Autodesk Fusion 360 part; units mm, degrees
(part 3 of 3)
  arc A127 (-91.1567, -68.8169) -> (-88.1567, -65.8169) centre (-91.1567, -65.8169) ccw
  line L128 (-91.1567, -127.2613) -> (-95.1567, -127.2613)
  arc A128 (-98.1567, -124.2613) -> (-95.1567, -127.2613) centre (-95.1567, -124.2613) ccw
  line L129 (-98.1567, -124.2613) -> (-98.1567, -120.2613)
  arc A129 (-95.1567, -117.2613) -> (-98.1567, -120.2613) centre (-95.1567, -120.2613) ccw
  line L130 (-95.1567, -117.2613) -> (-91.1567, -117.2613)
  arc A130 (-88.1567, -120.2613) -> (-91.1567, -117.2613) centre (-91.1567, -120.2613) ccw
  line L131 (-88.1567, -120.2613) -> (-88.1567, -124.2613)
  arc A131 (-91.1567, -127.2613) -> (-88.1567, -124.2613) centre (-91.1567, -124.2613) ccw
  line L132 (-120.3789, -156.4835) -> (-124.3789, -156.4835)
  arc A132 (-127.3789, -153.4835) -> (-124.3789, -156.4835) centre (-124.3789, -153.4835) ccw
  line L133 (-127.3789, -153.4835) -> (-127.3789, -149.4835)
  arc A133 (-124.3789, -146.4835) -> (-127.3789, -149.4835) centre (-124.3789, -149.4835) ccw
  line L134 (-124.3789, -146.4835) -> (-120.3789, -146.4835)
  arc A134 (-117.3789, -149.4835) -> (-120.3789, -146.4835) centre (-120.3789, -149.4835) ccw
  line L135 (-117.3789, -149.4835) -> (-117.3789, -153.4835)
  arc A135 (-120.3789, -156.4835) -> (-117.3789, -153.4835) centre (-120.3789, -153.4835) ccw
  line L136 (-105.7678, -141.8724) -> (-109.7678, -141.8724)
  arc A136 (-112.7678, -138.8724) -> (-109.7678, -141.8724) centre (-109.7678, -138.8724) ccw
  line L137 (-112.7678, -138.8724) -> (-112.7678, -134.8724)
  arc A137 (-109.7678, -131.8724) -> (-112.7678, -134.8724) centre (-109.7678, -134.8724) ccw
  line L138 (-109.7678, -131.8724) -> (-105.7678, -131.8724)
  arc A138 (-102.7678, -134.8724) -> (-105.7678, -131.8724) centre (-105.7678, -134.8724) ccw
  line L139 (-102.7678, -134.8724) -> (-102.7678, -138.8724)
  arc A139 (-105.7678, -141.8724) -> (-102.7678, -138.8724) centre (-105.7678, -138.8724) ccw
  line L140 (-134.99, -156.4835) -> (-138.99, -156.4835)
  arc A140 (-141.99, -153.4835) -> (-138.99, -156.4835) centre (-138.99, -153.4835) ccw
  line L141 (-141.99, -153.4835) -> (-141.99, -149.4835)
  arc A141 (-138.99, -146.4835) -> (-141.99, -149.4835) centre (-138.99, -149.4835) ccw
  line L142 (-138.99, -146.4835) -> (-134.99, -146.4835)
  arc A142 (-131.99, -149.4835) -> (-134.99, -146.4835) centre (-134.99, -149.4835) ccw
  line L143 (-131.99, -149.4835) -> (-131.99, -153.4835)
  arc A143 (-134.99, -156.4835) -> (-131.99, -153.4835) centre (-134.99, -153.4835) ccw
  line L144 (-120.3789, -39.5946) -> (-124.3789, -39.5946)
  arc A144 (-127.3789, -36.5946) -> (-124.3789, -39.5946) centre (-124.3789, -36.5946) ccw
  line L145 (-127.3789, -36.5946) -> (-127.3789, -32.5946)
  arc A145 (-124.3789, -29.5946) -> (-127.3789, -32.5946) centre (-124.3789, -32.5946) ccw
  line L146 (-124.3789, -29.5946) -> (-120.3789, -29.5946)
  arc A146 (-117.3789, -32.5946) -> (-120.3789, -29.5946) centre (-120.3789, -32.5946) ccw
  line L147 (-117.3789, -32.5946) -> (-117.3789, -36.5946)
  arc A147 (-120.3789, -39.5946) -> (-117.3789, -36.5946) centre (-120.3789, -36.5946) ccw
  line L148 (-134.99, -98.0391) -> (-138.99, -98.0391)
  arc A148 (-141.99, -95.0391) -> (-138.99, -98.0391) centre (-138.99, -95.0391) ccw
  line L149 (-141.99, -95.0391) -> (-141.99, -91.0391)
  arc A149 (-138.99, -88.0391) -> (-141.99, -91.0391) centre (-138.99, -91.0391) ccw
  line L150 (-138.99, -88.0391) -> (-134.99, -88.0391)
  arc A150 (-131.99, -91.0391) -> (-134.99, -88.0391) centre (-134.99, -91.0391) ccw
  line L151 (-131.99, -91.0391) -> (-131.99, -95.0391)
  arc A151 (-134.99, -98.0391) -> (-131.99, -95.0391) centre (-134.99, -95.0391) ccw
  line L152 (-164.2123, -68.8169) -> (-168.2123, -68.8169)
  arc A152 (-171.2123, -65.8169) -> (-168.2123, -68.8169) centre (-168.2123, -65.8169) ccw
  line L153 (-171.2123, -65.8169) -> (-171.2123, -61.8169)
  arc A153 (-168.2123, -58.8169) -> (-171.2123, -61.8169) centre (-168.2123, -61.8169) ccw
  line L154 (-168.2123, -58.8169) -> (-164.2123, -58.8169)
  arc A154 (-161.2123, -61.8169) -> (-164.2123, -58.8169) centre (-164.2123, -61.8169) ccw
  line L155 (-161.2123, -61.8169) -> (-161.2123, -65.8169)
  arc A155 (-164.2123, -68.8169) -> (-161.2123, -65.8169) centre (-164.2123, -65.8169) ccw
  line L156 (-91.1567, -141.8724) -> (-95.1567, -141.8724)
  arc A156 (-98.1567, -138.8724) -> (-95.1567, -141.8724) centre (-95.1567, -138.8724) ccw
  line L157 (-98.1567, -138.8724) -> (-98.1567, -134.8724)
  arc A157 (-95.1567, -131.8724) -> (-98.1567, -134.8724) centre (-95.1567, -134.8724) ccw
  line L158 (-95.1567, -131.8724) -> (-91.1567, -131.8724)
  arc A158 (-88.1567, -134.8724) -> (-91.1567, -131.8724) centre (-91.1567, -134.8724) ccw
  line L159 (-88.1567, -134.8724) -> (-88.1567, -138.8724)
  arc A159 (-91.1567, -141.8724) -> (-88.1567, -138.8724) centre (-91.1567, -138.8724) ccw
  line L160 (-149.6011, -112.6502) -> (-153.6011, -112.6502)
  arc A160 (-156.6011, -109.6502) -> (-153.6011, -112.6502) centre (-153.6011, -109.6502) ccw
  line L161 (-156.6011, -109.6502) -> (-156.6011, -105.6502)
  arc A161 (-153.6011, -102.6502) -> (-156.6011, -105.6502) centre (-153.6011, -105.6502) ccw
  line L162 (-153.6011, -102.6502) -> (-149.6011, -102.6502)
  arc A162 (-146.6011, -105.6502) -> (-149.6011, -102.6502) centre (-149.6011, -105.6502) ccw
  line L163 (-146.6011, -105.6502) -> (-146.6011, -109.6502)
  arc A163 (-149.6011, -112.6502) -> (-146.6011, -109.6502) centre (-149.6011, -109.6502) ccw
  line L164 (-105.7678, -112.6502) -> (-109.7678, -112.6502)
  arc A164 (-112.7678, -109.6502) -> (-109.7678, -112.6502) centre (-109.7678, -109.6502) ccw
  line L165 (-112.7678, -109.6502) -> (-112.7678, -105.6502)
  arc A165 (-109.7678, -102.6502) -> (-112.7678, -105.6502) centre (-109.7678, -105.6502) ccw
  line L166 (-109.7678, -102.6502) -> (-105.7678, -102.6502)
  arc A166 (-102.7678, -105.6502) -> (-105.7678, -102.6502) centre (-105.7678, -105.6502) ccw
  line L167 (-102.7678, -105.6502) -> (-102.7678, -109.6502)
  arc A167 (-105.7678, -112.6502) -> (-102.7678, -109.6502) centre (-105.7678, -109.6502) ccw
  line L168 (-76.5456, -141.8724) -> (-80.5456, -141.8724)
  arc A168 (-83.5456, -138.8724) -> (-80.5456, -141.8724) centre (-80.5456, -138.8724) ccw
  line L169 (-83.5456, -138.8724) -> (-83.5456, -134.8724)
  arc A169 (-80.5456, -131.8724) -> (-83.5456, -134.8724) centre (-80.5456, -134.8724) ccw
  line L170 (-80.5456, -131.8724) -> (-76.5456, -131.8724)
  arc A170 (-73.5456, -134.8724) -> (-76.5456, -131.8724) centre (-76.5456, -134.8724) ccw
  line L171 (-73.5456, -134.8724) -> (-73.5456, -138.8724)
  arc A171 (-76.5456, -141.8724) -> (-73.5456, -138.8724) centre (-76.5456, -138.8724) ccw
  line L172 (-149.6011, -127.2613) -> (-153.6011, -127.2613)
  arc A172 (-156.6011, -124.2613) -> (-153.6011, -127.2613) centre (-153.6011, -124.2613) ccw
  line L173 (-156.6011, -124.2613) -> (-156.6011, -120.2613)
  arc A173 (-153.6011, -117.2613) -> (-156.6011, -120.2613) centre (-153.6011, -120.2613) ccw
  line L174 (-153.6011, -117.2613) -> (-149.6011, -117.2613)
  arc A174 (-146.6011, -120.2613) -> (-149.6011, -117.2613) centre (-149.6011, -120.2613) ccw
  line L175 (-146.6011, -120.2613) -> (-146.6011, -124.2613)
  arc A175 (-149.6011, -127.2613) -> (-146.6011, -124.2613) centre (-149.6011, -124.2613) ccw
  line L176 (-164.2123, -141.8724) -> (-168.2123, -141.8724)
  arc A176 (-171.2123, -138.8724) -> (-168.2123, -141.8724) centre (-168.2123, -138.8724) ccw
  line L177 (-171.2123, -138.8724) -> (-171.2123, -134.8724)
  arc A177 (-168.2123, -131.8724) -> (-171.2123, -134.8724) centre (-168.2123, -134.8724) ccw
  line L178 (-168.2123, -131.8724) -> (-164.2123, -131.8724)
  arc A178 (-161.2123, -134.8724) -> (-164.2123, -131.8724) centre (-164.2123, -134.8724) ccw
  line L179 (-161.2123, -134.8724) -> (-161.2123, -138.8724)
  arc A179 (-164.2123, -141.8724) -> (-161.2123, -138.8724) centre (-164.2123, -138.8724) ccw
  line L180 (-47.3234, -171.0946) -> (-51.3234, -171.0946)
  arc A180 (-54.3234, -168.0946) -> (-51.3234, -171.0946) centre (-51.3234, -168.0946) ccw
  line L181 (-54.3234, -168.0946) -> (-54.3234, -164.0946)
  arc A181 (-51.3234, -161.0946) -> (-54.3234, -164.0946) centre (-51.3234, -164.0946) ccw
  line L182 (-51.3234, -161.0946) -> (-47.3234, -161.0946)
  arc A182 (-44.3234, -164.0946) -> (-47.3234, -161.0946) centre (-47.3234, -164.0946) ccw
  line L183 (-44.3234, -164.0946) -> (-44.3234, -168.0946)
  arc A183 (-47.3234, -171.0946) -> (-44.3234, -168.0946) centre (-47.3234, -168.0946) ccw
  line L184 (-32.7123, -156.4835) -> (-36.7123, -156.4835)
  arc A184 (-39.7123, -153.4835) -> (-36.7123, -156.4835) centre (-36.7123, -153.4835) ccw
  line L185 (-39.7123, -153.4835) -> (-39.7123, -149.4835)
  arc A185 (-36.7123, -146.4835) -> (-39.7123, -149.4835) centre (-36.7123, -149.4835) ccw
  line L186 (-36.7123, -146.4835) -> (-32.7123, -146.4835)
  arc A186 (-29.7123, -149.4835) -> (-32.7123, -146.4835) centre (-32.7123, -149.4835) ccw
  line L187 (-29.7123, -149.4835) -> (-29.7123, -153.4835)
  arc A187 (-32.7123, -156.4835) -> (-29.7123, -153.4835) centre (-32.7123, -153.4835) ccw
  line L188 (-32.7123, -127.2613) -> (-36.7123, -127.2613)
  arc A188 (-39.7123, -124.2613) -> (-36.7123, -127.2613) centre (-36.7123, -124.2613) ccw
  line L189 (-39.7123, -124.2613) -> (-39.7123, -120.2613)
  arc A189 (-36.7123, -117.2613) -> (-39.7123, -120.2613) centre (-36.7123, -120.2613) ccw
  line L190 (-36.7123, -117.2613) -> (-32.7123, -117.2613)
  arc A190 (-29.7123, -120.2613) -> (-32.7123, -117.2613) centre (-32.7123, -120.2613) ccw
  line L191 (-29.7123, -120.2613) -> (-29.7123, -124.2613)
  arc A191 (-32.7123, -127.2613) -> (-29.7123, -124.2613) centre (-32.7123, -124.2613) ccw
  line L192 (-47.3234, -127.2613) -> (-51.3234, -127.2613)
  arc A192 (-54.3234, -124.2613) -> (-51.3234, -127.2613) centre (-51.3234, -124.2613) ccw
  line L193 (-54.3234, -124.2613) -> (-54.3234, -120.2613)
  arc A193 (-51.3234, -117.2613) -> (-54.3234, -120.2613) centre (-51.3234, -120.2613) ccw
  line L194 (-51.3234, -117.2613) -> (-47.3234, -117.2613)
  arc A194 (-44.3234, -120.2613) -> (-47.3234, -117.2613) centre (-47.3234, -120.2613) ccw
  line L195 (-44.3234, -120.2613) -> (-44.3234, -124.2613)
  arc A195 (-47.3234, -127.2613) -> (-44.3234, -124.2613) centre (-47.3234, -124.2613) ccw
  line L196 (-105.7678, -83.428) -> (-109.7678, -83.428)
  arc A196 (-112.7678, -80.428) -> (-109.7678, -83.428) centre (-109.7678, -80.428) ccw
  line L197 (-112.7678, -80.428) -> (-112.7678, -76.428)
  arc A197 (-109.7678, -73.428) -> (-112.7678, -76.428) centre (-109.7678, -76.428) ccw
  line L198 (-109.7678, -73.428) -> (-105.7678, -73.428)
  arc A198 (-102.7678, -76.428) -> (-105.7678, -73.428) centre (-105.7678, -76.428) ccw
  line L199 (-102.7678, -76.428) -> (-102.7678, -80.428)
  arc A199 (-105.7678, -83.428) -> (-102.7678, -80.428) centre (-105.7678, -80.428) ccw
  line L200 (-120.3789, -68.8169) -> (-124.3789, -68.8169)
  arc A200 (-127.3789, -65.8169) -> (-124.3789, -68.8169) centre (-124.3789, -65.8169) ccw
  line L201 (-127.3789, -65.8169) -> (-127.3789, -61.8169)
  arc A201 (-124.3789, -58.8169) -> (-127.3789, -61.8169) centre (-124.3789, -61.8169) ccw
  line L202 (-124.3789, -58.8169) -> (-120.3789, -58.8169)
  arc A202 (-117.3789, -61.8169) -> (-120.3789, -58.8169) centre (-120.3789, -61.8169) ccw
  line L203 (-117.3789, -61.8169) -> (-117.3789, -65.8169)
  arc A203 (-120.3789, -68.8169) -> (-117.3789, -65.8169) centre (-120.3789, -65.8169) ccw
  line L204 (-91.1567, -171.0946) -> (-95.1567, -171.0946)
  arc A204 (-98.1567, -168.0946) -> (-95.1567, -171.0946) centre (-95.1567, -168.0946) ccw
  line L205 (-98.1567, -168.0946) -> (-98.1567, -164.0946)
  arc A205 (-95.1567, -161.0946) -> (-98.1567, -164.0946) centre (-95.1567, -164.0946) ccw
  line L206 (-95.1567, -161.0946) -> (-91.1567, -161.0946)
  arc A206 (-88.1567, -164.0946) -> (-91.1567, -161.0946) centre (-91.1567, -164.0946) ccw
  line L207 (-88.1567, -164.0946) -> (-88.1567, -168.0946)
  arc A207 (-91.1567, -171.0946) -> (-88.1567, -168.0946) centre (-91.1567, -168.0946) ccw
  line L208 (-47.3234, -156.4835) -> (-51.3234, -156.4835)
  arc A208 (-54.3234, -153.4835) -> (-51.3234, -156.4835) centre (-51.3234, -153.4835) ccw
  line L209 (-54.3234, -153.4835) -> (-54.3234, -149.4835)
  arc A209 (-51.3234, -146.4835) -> (-54.3234, -149.4835) centre (-51.3234, -149.4835) ccw
  line L210 (-51.3234, -146.4835) -> (-47.3234, -146.4835)
  arc A210 (-44.3234, -149.4835) -> (-47.3234, -146.4835) centre (-47.3234, -149.4835) ccw
  line L211 (-44.3234, -149.4835) -> (-44.3234, -153.4835)
  arc A211 (-47.3234, -156.4835) -> (-44.3234, -153.4835) centre (-47.3234, -153.4835) ccw
  line L212 (-134.99, -39.5946) -> (-138.99, -39.5946)
  arc A212 (-141.99, -36.5946) -> (-138.99, -39.5946) centre (-138.99, -36.5946) ccw
  line L213 (-141.99, -36.5946) -> (-141.99, -32.5946)
  arc A213 (-138.99, -29.5946) -> (-141.99, -32.5946) centre (-138.99, -32.5946) ccw
  line L214 (-138.99, -29.5946) -> (-134.99, -29.5946)
  arc A214 (-131.99, -32.5946) -> (-134.99, -29.5946) centre (-134.99, -32.5946) ccw
  line L215 (-131.99, -32.5946) -> (-131.99, -36.5946)
  arc A215 (-134.99, -39.5946) -> (-131.99, -36.5946) centre (-134.99, -36.5946) ccw
  line L216 (-134.99, -141.8724) -> (-138.99, -141.8724)
  arc A216 (-141.99, -138.8724) -> (-138.99, -141.8724) centre (-138.99, -138.8724) ccw
  line L217 (-141.99, -138.8724) -> (-141.99, -134.8724)
  arc A217 (-138.99, -131.8724) -> (-141.99, -134.8724) centre (-138.99, -134.8724) ccw
  line L218 (-138.99, -131.8724) -> (-134.99, -131.8724)
  arc A218 (-131.99, -134.8724) -> (-134.99, -131.8724) centre (-134.99, -134.8724) ccw
  line L219 (-131.99, -134.8724) -> (-131.99, -138.8724)
  arc A219 (-134.99, -141.8724) -> (-131.99, -138.8724) centre (-134.99, -138.8724) ccw
  line L220 (-120.3789, -127.2613) -> (-124.3789, -127.2613)
  arc A220 (-127.3789, -124.2613) -> (-124.3789, -127.2613) centre (-124.3789, -124.2613) ccw
  line L221 (-127.3789, -124.2613) -> (-127.3789, -120.2613)
  arc A221 (-124.3789, -117.2613) -> (-127.3789, -120.2613) centre (-124.3789, -120.2613) ccw
  line L222 (-124.3789, -117.2613) -> (-120.3789, -117.2613)
  arc A222 (-117.3789, -120.2613) -> (-120.3789, -117.2613) centre (-120.3789, -120.2613) ccw
  line L223 (-117.3789, -120.2613) -> (-117.3789, -124.2613)
  arc A223 (-120.3789, -127.2613) -> (-117.3789, -124.2613) centre (-120.3789, -124.2613) ccw
  line L224 (-164.2123, -127.2613) -> (-168.2123, -127.2613)
  arc A224 (-171.2123, -124.2613) -> (-168.2123, -127.2613) centre (-168.2123, -124.2613) ccw
  line L225 (-171.2123, -124.2613) -> (-171.2123, -120.2613)
  arc A225 (-168.2123, -117.2613) -> (-171.2123, -120.2613) centre (-168.2123, -120.2613) ccw
  line L226 (-168.2123, -117.2613) -> (-164.2123, -117.2613)
  arc A226 (-161.2123, -120.2613) -> (-164.2123, -117.2613) centre (-164.2123, -120.2613) ccw
  line L227 (-161.2123, -120.2613) -> (-161.2123, -124.2613)
  arc A227 (-164.2123, -127.2613) -> (-161.2123, -124.2613) centre (-164.2123, -124.2613) ccw
  line L228 (-134.99, -68.8169) -> (-138.99, -68.8169)
  arc A228 (-141.99, -65.8169) -> (-138.99, -68.8169) centre (-138.99, -65.8169) ccw
  line L229 (-141.99, -65.8169) -> (-141.99, -61.8169)
  arc A229 (-138.99, -58.8169) -> (-141.99, -61.8169) centre (-138.99, -61.8169) ccw
  line L230 (-138.99, -58.8169) -> (-134.99, -58.8169)
  arc A230 (-131.99, -61.8169) -> (-134.99, -58.8169) centre (-134.99, -61.8169) ccw
  line L231 (-131.99, -61.8169) -> (-131.99, -65.8169)
  arc A231 (-134.99, -68.8169) -> (-131.99, -65.8169) centre (-134.99, -65.8169) ccw
  line L232 (-32.7123, -171.0946) -> (-36.7123, -171.0946)
  arc A232 (-39.7123, -168.0946) -> (-36.7123, -171.0946) centre (-36.7123, -168.0946) ccw
  line L233 (-39.7123, -168.0946) -> (-39.7123, -164.0946)
  arc A233 (-36.7123, -161.0946) -> (-39.7123, -164.0946) centre (-36.7123, -164.0946) ccw
  line L234 (-36.7123, -161.0946) -> (-32.7123, -161.0946)
  arc A234 (-29.7123, -164.0946) -> (-32.7123, -161.0946) centre (-32.7123, -164.0946) ccw
  line L235 (-29.7123, -164.0946) -> (-29.7123, -168.0946)
  arc A235 (-32.7123, -171.0946) -> (-29.7123, -168.0946) centre (-32.7123, -168.0946) ccw
  line L236 (-105.7678, -54.2058) -> (-109.7678, -54.2058)
  arc A236 (-112.7678, -51.2058) -> (-109.7678, -54.2058) centre (-109.7678, -51.2058) ccw
  line L237 (-112.7678, -51.2058) -> (-112.7678, -47.2058)
  arc A237 (-109.7678, -44.2058) -> (-112.7678, -47.2058) centre (-109.7678, -47.2058) ccw
  line L238 (-109.7678, -44.2058) -> (-105.7678, -44.2058)
  arc A238 (-102.7678, -47.2058) -> (-105.7678, -44.2058) centre (-105.7678, -47.2058) ccw
  line L239 (-102.7678, -47.2058) -> (-102.7678, -51.2058)
  arc A239 (-105.7678, -54.2058) -> (-102.7678, -51.2058) centre (-105.7678, -51.2058) ccw
  line L240 (-61.9345, -171.0946) -> (-65.9345, -171.0946)
  arc A240 (-68.9345, -168.0946) -> (-65.9345, -171.0946) centre (-65.9345, -168.0946) ccw
  line L241 (-68.9345, -168.0946) -> (-68.9345, -164.0946)
  arc A241 (-65.9345, -161.0946) -> (-68.9345, -164.0946) centre (-65.9345, -164.0946) ccw
  line L242 (-65.9345, -161.0946) -> (-61.9345, -161.0946)
  arc A242 (-58.9345, -164.0946) -> (-61.9345, -161.0946) centre (-61.9345, -164.0946) ccw
  line L243 (-58.9345, -164.0946) -> (-58.9345, -168.0946)
  arc A243 (-61.9345, -171.0946) -> (-58.9345, -168.0946) centre (-61.9345, -168.0946) ccw
  line L244 (-47.3234, -141.8724) -> (-51.3234, -141.8724)
  arc A244 (-54.3234, -138.8724) -> (-51.3234, -141.8724) centre (-51.3234, -138.8724) ccw
  line L245 (-54.3234, -138.8724) -> (-54.3234, -134.8724)
  arc A245 (-51.3234, -131.8724) -> (-54.3234, -134.8724) centre (-51.3234, -134.8724) ccw
  line L246 (-51.3234, -131.8724) -> (-47.3234, -131.8724)
  arc A246 (-44.3234, -134.8724) -> (-47.3234, -131.8724) centre (-47.3234, -134.8724) ccw
  line L247 (-44.3234, -134.8724) -> (-44.3234, -138.8724)
  arc A247 (-47.3234, -141.8724) -> (-44.3234, -138.8724) centre (-47.3234, -138.8724) ccw
  line L248 (-149.6011, -98.0391) -> (-153.6011, -98.0391)
  arc A248 (-156.6011, -95.0391) -> (-153.6011, -98.0391) centre (-153.6011, -95.0391) ccw
  line L249 (-156.6011, -95.0391) -> (-156.6011, -91.0391)
  arc A249 (-153.6011, -88.0391) -> (-156.6011, -91.0391) centre (-153.6011, -91.0391) ccw
  line L250 (-153.6011, -88.0391) -> (-149.6011, -88.0391)
  arc A250 (-146.6011, -91.0391) -> (-149.6011, -88.0391) centre (-149.6011, -91.0391) ccw
  line L251 (-146.6011, -91.0391) -> (-146.6011, -95.0391)
  arc A251 (-149.6011, -98.0391) -> (-146.6011, -95.0391) centre (-149.6011, -95.0391) ccw
  line L252 (-149.6011, -54.2058) -> (-153.6011, -54.2058)
  arc A252 (-156.6011, -51.2058) -> (-153.6011, -54.2058) centre (-153.6011, -51.2058) ccw
  line L253 (-156.6011, -51.2058) -> (-156.6011, -47.2058)
  arc A253 (-153.6011, -44.2058) -> (-156.6011, -47.2058) centre (-153.6011, -47.2058) ccw
  line L254 (-153.6011, -44.2058) -> (-149.6011, -44.2058)
  arc A254 (-146.6011, -47.2058) -> (-149.6011, -44.2058) centre (-149.6011, -47.2058) ccw
  line L255 (-146.6011, -47.2058) -> (-146.6011, -51.2058)
  arc A255 (-149.6011, -54.2058) -> (-146.6011, -51.2058) centre (-149.6011, -51.2058) ccw
  line L256 (-105.7678, -156.4835) -> (-109.7678, -156.4835)
  arc A256 (-112.7678, -153.4835) -> (-109.7678, -156.4835) centre (-109.7678, -153.4835) ccw
  line L257 (-112.7678, -153.4835) -> (-112.7678, -149.4835)
  arc A257 (-109.7678, -146.4835) -> (-112.7678, -149.4835) centre (-109.7678, -149.4835) ccw
  line L258 (-109.7678, -146.4835) -> (-105.7678, -146.4835)
  arc A258 (-102.7678, -149.4835) -> (-105.7678, -146.4835) centre (-105.7678, -149.4835) ccw
  line L259 (-102.7678, -149.4835) -> (-102.7678, -153.4835)
  arc A259 (-105.7678, -156.4835) -> (-102.7678, -153.4835) centre (-105.7678, -153.4835) ccw
  line L260 (-164.2123, -171.0946) -> (-168.2123, -171.0946)
  arc A260 (-171.2123, -168.0946) -> (-168.2123, -171.0946) centre (-168.2123, -168.0946) ccw
  line L261 (-171.2123, -168.0946) -> (-171.2123, -164.0946)
  arc A261 (-168.2123, -161.0946) -> (-171.2123, -164.0946) centre (-168.2123, -164.0946) ccw
  line L262 (-168.2123, -161.0946) -> (-164.2123, -161.0946)
  arc A262 (-161.2123, -164.0946) -> (-164.2123, -161.0946) centre (-164.2123, -164.0946) ccw
  line L263 (-161.2123, -164.0946) -> (-161.2123, -168.0946)
  arc A263 (-164.2123, -171.0946) -> (-161.2123, -168.0946) centre (-164.2123, -168.0946) ccw
  line L264 (-149.6011, -171.0946) -> (-153.6011, -171.0946)
  arc A264 (-156.6011, -168.0946) -> (-153.6011, -171.0946) centre (-153.6011, -168.0946) ccw
  line L265 (-156.6011, -168.0946) -> (-156.6011, -164.0946)
  arc A265 (-153.6011, -161.0946) -> (-156.6011, -164.0946) centre (-153.6011, -164.0946) ccw
  line L266 (-153.6011, -161.0946) -> (-149.6011, -161.0946)
  arc A266 (-146.6011, -164.0946) -> (-149.6011, -161.0946) centre (-149.6011, -164.0946) ccw
  line L267 (-146.6011, -164.0946) -> (-146.6011, -168.0946)
  arc A267 (-149.6011, -171.0946) -> (-146.6011, -168.0946) centre (-149.6011, -168.0946) ccw
  line L268 (-91.1567, -83.428) -> (-95.1567, -83.428)
  arc A268 (-98.1567, -80.428) -> (-95.1567, -83.428) centre (-95.1567, -80.428) ccw
  line L269 (-98.1567, -80.428) -> (-98.1567, -76.428)
  arc A269 (-95.1567, -73.428) -> (-98.1567, -76.428) centre (-95.1567, -76.428) ccw
  line L270 (-95.1567, -73.428) -> (-91.1567, -73.428)
  arc A270 (-88.1567, -76.428) -> (-91.1567, -73.428) centre (-91.1567, -76.428) ccw
  line L271 (-88.1567, -76.428) -> (-88.1567, -80.428)
  arc A271 (-91.1567, -83.428) -> (-88.1567, -80.428) centre (-91.1567, -80.428) ccw
  line L272 (-47.3234, -68.8169) -> (-51.3234, -68.8169)
  arc A272 (-54.3234, -65.8169) -> (-51.3234, -68.8169) centre (-51.3234, -65.8169) ccw
  line L273 (-54.3234, -65.8169) -> (-54.3234, -61.8169)
  arc A273 (-51.3234, -58.8169) -> (-54.3234, -61.8169) centre (-51.3234, -61.8169) ccw
  line L274 (-51.3234, -58.8169) -> (-47.3234, -58.8169)
  arc A274 (-44.3234, -61.8169) -> (-47.3234, -58.8169) centre (-47.3234, -61.8169) ccw
  line L275 (-44.3234, -61.8169) -> (-44.3234, -65.8169)
  arc A275 (-47.3234, -68.8169) -> (-44.3234, -65.8169) centre (-47.3234, -65.8169) ccw
  line L276 (-32.7123, -54.2058) -> (-36.7123, -54.2058)
  arc A276 (-39.7123, -51.2058) -> (-36.7123, -54.2058) centre (-36.7123, -51.2058) ccw
  line L277 (-39.7123, -51.2058) -> (-39.7123, -47.2058)
  arc A277 (-36.7123, -44.2058) -> (-39.7123, -47.2058) centre (-36.7123, -47.2058) ccw
  line L278 (-36.7123, -44.2058) -> (-32.7123, -44.2058)
  arc A278 (-29.7123, -47.2058) -> (-32.7123, -44.2058) centre (-32.7123, -47.2058) ccw
  line L279 (-29.7123, -47.2058) -> (-29.7123, -51.2058)
  arc A279 (-32.7123, -54.2058) -> (-29.7123, -51.2058) centre (-32.7123, -51.2058) ccw
  line L280 (-32.7123, -39.5946) -> (-36.7123, -39.5946)
  arc A280 (-39.7123, -36.5946) -> (-36.7123, -39.5946) centre (-36.7123, -36.5946) ccw
  line L281 (-39.7123, -36.5946) -> (-39.7123, -32.5946)
  arc A281 (-36.7123, -29.5946) -> (-39.7123, -32.5946) centre (-36.7123, -32.5946) ccw
  line L282 (-36.7123, -29.5946) -> (-32.7123, -29.5946)
  arc A282 (-29.7123, -32.5946) -> (-32.7123, -29.5946) centre (-32.7123, -32.5946) ccw
  line L283 (-29.7123, -32.5946) -> (-29.7123, -36.5946)
  arc A283 (-32.7123, -39.5946) -> (-29.7123, -36.5946) centre (-32.7123, -36.5946) ccw
  line L284 (-91.1567, -39.5946) -> (-95.1567, -39.5946)
  arc A284 (-98.1567, -36.5946) -> (-95.1567, -39.5946) centre (-95.1567, -36.5946) ccw
  line L285 (-98.1567, -36.5946) -> (-98.1567, -32.5946)
  arc A285 (-95.1567, -29.5946) -> (-98.1567, -32.5946) centre (-95.1567, -32.5946) ccw
  line L286 (-95.1567, -29.5946) -> (-91.1567, -29.5946)
  arc A286 (-88.1567, -32.5946) -> (-91.1567, -29.5946) centre (-91.1567, -32.5946) ccw
  line L287 (-88.1567, -32.5946) -> (-88.1567, -36.5946)
  arc A287 (-91.1567, -39.5946) -> (-88.1567, -36.5946) centre (-91.1567, -36.5946) ccw
  line L288 (-61.9345, -98.0391) -> (-65.9345, -98.0391)
  arc A288 (-68.9345, -95.0391) -> (-65.9345, -98.0391) centre (-65.9345, -95.0391) ccw
  line L289 (-68.9345, -95.0391) -> (-68.9345, -91.0391)
  arc A289 (-65.9345, -88.0391) -> (-68.9345, -91.0391) centre (-65.9345, -91.0391) ccw
  line L290 (-65.9345, -88.0391) -> (-61.9345, -88.0391)
  arc A290 (-58.9345, -91.0391) -> (-61.9345, -88.0391) centre (-61.9345, -91.0391) ccw
  line L291 (-58.9345, -91.0391) -> (-58.9345, -95.0391)
  arc A291 (-61.9345, -98.0391) -> (-58.9345, -95.0391) centre (-61.9345, -95.0391) ccw
  line L292 (-32.7123, -98.0391) -> (-36.7123, -98.0391)
  arc A292 (-39.7123, -95.0391) -> (-36.7123, -98.0391) centre (-36.7123, -95.0391) ccw
  line L293 (-39.7123, -95.0391) -> (-39.7123, -91.0391)
  arc A293 (-36.7123, -88.0391) -> (-39.7123, -91.0391) centre (-36.7123, -91.0391) ccw
  line L294 (-36.7123, -88.0391) -> (-32.7123, -88.0391)
  arc A294 (-29.7123, -91.0391) -> (-32.7123, -88.0391) centre (-32.7123, -91.0391) ccw
  line L295 (-29.7123, -91.0391) -> (-29.7123, -95.0391)
  arc A295 (-32.7123, -98.0391) -> (-29.7123, -95.0391) centre (-32.7123, -95.0391) ccw
  line L296 (-61.9345, -112.6502) -> (-65.9345, -112.6502)
  arc A296 (-68.9345, -109.6502) -> (-65.9345, -112.6502) centre (-65.9345, -109.6502) ccw
  line L297 (-68.9345, -109.6502) -> (-68.9345, -105.6502)
  arc A297 (-65.9345, -102.6502) -> (-68.9345, -105.6502) centre (-65.9345, -105.6502) ccw
  line L298 (-65.9345, -102.6502) -> (-61.9345, -102.6502)
  arc A298 (-58.9345, -105.6502) -> (-61.9345, -102.6502) centre (-61.9345, -105.6502) ccw
  line L299 (-58.9345, -105.6502) -> (-58.9345, -109.6502)
  arc A299 (-61.9345, -112.6502) -> (-58.9345, -109.6502) centre (-61.9345, -109.6502) ccw
  line L300 (-91.1567, -112.6502) -> (-95.1567, -112.6502)
  arc A300 (-98.1567, -109.6502) -> (-95.1567, -112.6502) centre (-95.1567, -109.6502) ccw
  line L301 (-98.1567, -109.6502) -> (-98.1567, -105.6502)
  arc A301 (-95.1567, -102.6502) -> (-98.1567, -105.6502) centre (-95.1567, -105.6502) ccw
  line L302 (-95.1567, -102.6502) -> (-91.1567, -102.6502)
  arc A302 (-88.1567, -105.6502) -> (-91.1567, -102.6502) centre (-91.1567, -105.6502) ccw
  line L303 (-88.1567, -105.6502) -> (-88.1567, -109.6502)
  arc A303 (-91.1567, -112.6502) -> (-88.1567, -109.6502) centre (-91.1567, -109.6502) ccw
  line L304 (-76.5456, -98.0391) -> (-80.5456, -98.0391)
  arc A304 (-83.5456, -95.0391) -> (-80.5456, -98.0391) centre (-80.5456, -95.0391) ccw
  line L305 (-83.5456, -95.0391) -> (-83.5456, -91.0391)
  arc A305 (-80.5456, -88.0391) -> (-83.5456, -91.0391) centre (-80.5456, -91.0391) ccw
  line L306 (-80.5456, -88.0391) -> (-76.5456, -88.0391)
  arc A306 (-73.5456, -91.0391) -> (-76.5456, -88.0391) centre (-76.5456, -91.0391) ccw
  line L307 (-73.5456, -91.0391) -> (-73.5456, -95.0391)
  arc A307 (-76.5456, -98.0391) -> (-73.5456, -95.0391) centre (-76.5456, -95.0391) ccw
  line L308 (-61.9345, -39.5946) -> (-65.9345, -39.5946)
  arc A308 (-68.9345, -36.5946) -> (-65.9345, -39.5946) centre (-65.9345, -36.5946) ccw
  line L309 (-68.9345, -36.5946) -> (-68.9345, -32.5946)
  arc A309 (-65.9345, -29.5946) -> (-68.9345, -32.5946) centre (-65.9345, -32.5946) ccw
  line L310 (-65.9345, -29.5946) -> (-61.9345, -29.5946)
  arc A310 (-58.9345, -32.5946) -> (-61.9345, -29.5946) centre (-61.9345, -32.5946) ccw
  line L311 (-58.9345, -32.5946) -> (-58.9345, -36.5946)
  arc A311 (-61.9345, -39.5946) -> (-58.9345, -36.5946) centre (-61.9345, -36.5946) ccw
  line L312 (-61.9345, -54.2058) -> (-65.9345, -54.2058)
  arc A312 (-68.9345, -51.2058) -> (-65.9345, -54.2058) centre (-65.9345, -51.2058) ccw
  line L313 (-68.9345, -51.2058) -> (-68.9345, -47.2058)
  arc A313 (-65.9345, -44.2058) -> (-68.9345, -47.2058) centre (-65.9345, -47.2058) ccw
  line L314 (-65.9345, -44.2058) -> (-61.9345, -44.2058)
  arc A314 (-58.9345, -47.2058) -> (-61.9345, -44.2058) centre (-61.9345, -47.2058) ccw
  line L315 (-58.9345, -47.2058) -> (-58.9345, -51.2058)
  arc A315 (-61.9345, -54.2058) -> (-58.9345, -51.2058) centre (-61.9345, -51.2058) ccw
  line L316 (-47.3234, -54.2058) -> (-51.3234, -54.2058)
  arc A316 (-54.3234, -51.2058) -> (-51.3234, -54.2058) centre (-51.3234, -51.2058) ccw
  line L317 (-54.3234, -51.2058) -> (-54.3234, -47.2058)
  arc A317 (-51.3234, -44.2058) -> (-54.3234, -47.2058) centre (-51.3234, -47.2058) ccw
  line L318 (-51.3234, -44.2058) -> (-47.3234, -44.2058)
  arc A318 (-44.3234, -47.2058) -> (-47.3234, -44.2058) centre (-47.3234, -47.2058) ccw
  line L319 (-44.3234, -47.2058) -> (-44.3234, -51.2058)
  arc A319 (-47.3234, -54.2058) -> (-44.3234, -51.2058) centre (-47.3234, -51.2058) ccw
  line L320 (-61.9345, -83.428) -> (-65.9345, -83.428)
  arc A320 (-68.9345, -80.428) -> (-65.9345, -83.428) centre (-65.9345, -80.428) ccw
  line L321 (-68.9345, -80.428) -> (-68.9345, -76.428)
  arc A321 (-65.9345, -73.428) -> (-68.9345, -76.428) centre (-65.9345, -76.428) ccw
  line L322 (-65.9345, -73.428) -> (-61.9345, -73.428)
  arc A322 (-58.9345, -76.428) -> (-61.9345, -73.428) centre (-61.9345, -76.428) ccw
  line L323 (-58.9345, -76.428) -> (-58.9345, -80.428)
  arc A323 (-61.9345, -83.428) -> (-58.9345, -80.428) centre (-61.9345, -80.428) ccw
  line L324 (-32.7123, -68.8169) -> (-36.7123, -68.8169)
  arc A324 (-39.7123, -65.8169) -> (-36.7123, -68.8169) centre (-36.7123, -65.8169) ccw
  line L325 (-39.7123, -65.8169) -> (-39.7123, -61.8169)
  arc A325 (-36.7123, -58.8169) -> (-39.7123, -61.8169) centre (-36.7123, -61.8169) ccw
  line L326 (-36.7123, -58.8169) -> (-32.7123, -58.8169)
  arc A326 (-29.7123, -61.8169) -> (-32.7123, -58.8169) centre (-32.7123, -61.8169) ccw
  line L327 (-29.7123, -61.8169) -> (-29.7123, -65.8169)
  arc A327 (-32.7123, -68.8169) -> (-29.7123, -65.8169) centre (-32.7123, -65.8169) ccw
  line L328 (-149.6011, -156.4835) -> (-153.6011, -156.4835)
  arc A328 (-156.6011, -153.4835) -> (-153.6011, -156.4835) centre (-153.6011, -153.4835) ccw
  line L329 (-156.6011, -153.4835) -> (-156.6011, -149.4835)
  arc A329 (-153.6011, -146.4835) -> (-156.6011, -149.4835) centre (-153.6011, -149.4835) ccw
  line L330 (-153.6011, -146.4835) -> (-149.6011, -146.4835)
  arc A330 (-146.6011, -149.4835) -> (-149.6011, -146.4835) centre (-149.6011, -149.4835) ccw
  line L331 (-146.6011, -149.4835) -> (-146.6011, -153.4835)
  arc A331 (-149.6011, -156.4835) -> (-146.6011, -153.4835) centre (-149.6011, -153.4835) ccw
  line L332 (-120.3789, -141.8724) -> (-124.3789, -141.8724)
  arc A332 (-127.3789, -138.8724) -> (-124.3789, -141.8724) centre (-124.3789, -138.8724) ccw
  line L333 (-127.3789, -138.8724) -> (-127.3789, -134.8724)
  arc A333 (-124.3789, -131.8724) -> (-127.3789, -134.8724) centre (-124.3789, -134.8724) ccw
  line L334 (-124.3789, -131.8724) -> (-120.3789, -131.8724)
  arc A334 (-117.3789, -134.8724) -> (-120.3789, -131.8724) centre (-120.3789, -134.8724) ccw
  line L335 (-117.3789, -134.8724) -> (-117.3789, -138.8724)
  arc A335 (-120.3789, -141.8724) -> (-117.3789, -138.8724) centre (-120.3789, -138.8724) ccw
  line L336 (-105.7678, -171.0946) -> (-109.7678, -171.0946)
  arc A336 (-112.7678, -168.0946) -> (-109.7678, -171.0946) centre (-109.7678, -168.0946) ccw
  line L337 (-112.7678, -168.0946) -> (-112.7678, -164.0946)
  arc A337 (-109.7678, -161.0946) -> (-112.7678, -164.0946) centre (-109.7678, -164.0946) ccw
  line L338 (-109.7678, -161.0946) -> (-105.7678, -161.0946)
  arc A338 (-102.7678, -164.0946) -> (-105.7678, -161.0946) centre (-105.7678, -164.0946) ccw
  line L339 (-102.7678, -164.0946) -> (-102.7678, -168.0946)
  arc A339 (-105.7678, -171.0946) -> (-102.7678, -168.0946) centre (-105.7678, -168.0946) ccw
  line L340 (-149.6011, -39.5946) -> (-153.6011, -39.5946)
  arc A340 (-156.6011, -36.5946) -> (-153.6011, -39.5946) centre (-153.6011, -36.5946) ccw
  line L341 (-156.6011, -36.5946) -> (-156.6011, -32.5946)
  arc A341 (-153.6011, -29.5946) -> (-156.6011, -32.5946) centre (-153.6011, -32.5946) ccw
  line L342 (-153.6011, -29.5946) -> (-149.6011, -29.5946)
  arc A342 (-146.6011, -32.5946) -> (-149.6011, -29.5946) centre (-149.6011, -32.5946) ccw
  line L343 (-146.6011, -32.5946) -> (-146.6011, -36.5946)
  arc A343 (-149.6011, -39.5946) -> (-146.6011, -36.5946) centre (-149.6011, -36.5946) ccw
  line L344 (-61.9345, -141.8724) -> (-65.9345, -141.8724)
  arc A344 (-68.9345, -138.8724) -> (-65.9345, -141.8724) centre (-65.9345, -138.8724) ccw
  line L345 (-68.9345, -138.8724) -> (-68.9345, -134.8724)
  arc A345 (-65.9345, -131.8724) -> (-68.9345, -134.8724) centre (-65.9345, -134.8724) ccw
  line L346 (-65.9345, -131.8724) -> (-61.9345, -131.8724)
  arc A346 (-58.9345, -134.8724) -> (-61.9345, -131.8724) centre (-61.9345, -134.8724) ccw
  line L347 (-58.9345, -134.8724) -> (-58.9345, -138.8724)
  arc A347 (-61.9345, -141.8724) -> (-58.9345, -138.8724) centre (-61.9345, -138.8724) ccw
  line L348 (-61.9345, -127.2613) -> (-65.9345, -127.2613)
  arc A348 (-68.9345, -124.2613) -> (-65.9345, -127.2613) centre (-65.9345, -124.2613) ccw
  line L349 (-68.9345, -124.2613) -> (-68.9345, -120.2613)
  arc A349 (-65.9345, -117.2613) -> (-68.9345, -120.2613) centre (-65.9345, -120.2613) ccw
  line L350 (-65.9345, -117.2613) -> (-61.9345, -117.2613)
  arc A350 (-58.9345, -120.2613) -> (-61.9345, -117.2613) centre (-61.9345, -120.2613) ccw
  line L351 (-58.9345, -120.2613) -> (-58.9345, -124.2613)
  arc A351 (-61.9345, -127.2613) -> (-58.9345, -124.2613) centre (-61.9345, -124.2613) ccw
  line L352 (-164.2123, -112.6502) -> (-168.2123, -112.6502)
  arc A352 (-171.2123, -109.6502) -> (-168.2123, -112.6502) centre (-168.2123, -109.6502) ccw
  line L353 (-171.2123, -109.6502) -> (-171.2123, -105.6502)
  arc A353 (-168.2123, -102.6502) -> (-171.2123, -105.6502) centre (-168.2123, -105.6502) ccw
  line L354 (-168.2123, -102.6502) -> (-164.2123, -102.6502)
  arc A354 (-161.2123, -105.6502) -> (-164.2123, -102.6502) centre (-164.2123, -105.6502) ccw
  line L355 (-161.2123, -105.6502) -> (-161.2123, -109.6502)
  arc A355 (-164.2123, -112.6502) -> (-161.2123, -109.6502) centre (-164.2123, -109.6502) ccw
  line L356 (-105.7678, -39.5946) -> (-109.7678, -39.5946)
  arc A356 (-112.7678, -36.5946) -> (-109.7678, -39.5946) centre (-109.7678, -36.5946) ccw
  line L357 (-112.7678, -36.5946) -> (-112.7678, -32.5946)
  arc A357 (-109.7678, -29.5946) -> (-112.7678, -32.5946) centre (-109.7678, -32.5946) ccw
  line L358 (-109.7678, -29.5946) -> (-105.7678, -29.5946)
  arc A358 (-102.7678, -32.5946) -> (-105.7678, -29.5946) centre (-105.7678, -32.5946) ccw
  line L359 (-102.7678, -32.5946) -> (-102.7678, -36.5946)
  arc A359 (-105.7678, -39.5946) -> (-102.7678, -36.5946) centre (-105.7678, -36.5946) ccw
  line L360 (-164.2123, -83.428) -> (-168.2123, -83.428)
  arc A360 (-171.2123, -80.428) -> (-168.2123, -83.428) centre (-168.2123, -80.428) ccw
  line L361 (-171.2123, -80.428) -> (-171.2123, -76.428)
  arc A361 (-168.2123, -73.428) -> (-171.2123, -76.428) centre (-168.2123, -76.428) ccw
  line L362 (-168.2123, -73.428) -> (-164.2123, -73.428)
  arc A362 (-161.2123, -76.428) -> (-164.2123, -73.428) centre (-164.2123, -76.428) ccw
  line L363 (-161.2123, -76.428) -> (-161.2123, -80.428)
  arc A363 (-164.2123, -83.428) -> (-161.2123, -80.428) centre (-164.2123, -80.428) ccw
  line L364 (-61.9345, -156.4835) -> (-65.9345, -156.4835)
  arc A364 (-68.9345, -153.4835) -> (-65.9345, -156.4835) centre (-65.9345, -153.4835) ccw
  line L365 (-68.9345, -153.4835) -> (-68.9345, -149.4835)
  arc A365 (-65.9345, -146.4835) -> (-68.9345, -149.4835) centre (-65.9345, -149.4835) ccw
  line L366 (-65.9345, -146.4835) -> (-61.9345, -146.4835)
  arc A366 (-58.9345, -149.4835) -> (-61.9345, -146.4835) centre (-61.9345, -149.4835) ccw
  line L367 (-58.9345, -149.4835) -> (-58.9345, -153.4835)
  arc A367 (-61.9345, -156.4835) -> (-58.9345, -153.4835) centre (-61.9345, -153.4835) ccw
  line L368 (-120.3789, -112.6502) -> (-124.3789, -112.6502)
  arc A368 (-127.3789, -109.6502) -> (-124.3789, -112.6502) centre (-124.3789, -109.6502) ccw
  line L369 (-127.3789, -109.6502) -> (-127.3789, -105.6502)
  arc A369 (-124.3789, -102.6502) -> (-127.3789, -105.6502) centre (-124.3789, -105.6502) ccw
  line L370 (-124.3789, -102.6502) -> (-120.3789, -102.6502)
  arc A370 (-117.3789, -105.6502) -> (-120.3789, -102.6502) centre (-120.3789, -105.6502) ccw
  line L371 (-117.3789, -105.6502) -> (-117.3789, -109.6502)
  arc A371 (-120.3789, -112.6502) -> (-117.3789, -109.6502) centre (-120.3789, -109.6502) ccw
  line L372 (-134.99, -127.2613) -> (-138.99, -127.2613)
  arc A372 (-141.99, -124.2613) -> (-138.99, -127.2613) centre (-138.99, -124.2613) ccw
  line L373 (-141.99, -124.2613) -> (-141.99, -120.2613)
  arc A373 (-138.99, -117.2613) -> (-141.99, -120.2613) centre (-138.99, -120.2613) ccw
  line L374 (-138.99, -117.2613) -> (-134.99, -117.2613)
  arc A374 (-131.99, -120.2613) -> (-134.99, -117.2613) centre (-134.99, -120.2613) ccw
  line L375 (-131.99, -120.2613) -> (-131.99, -124.2613)
  arc A375 (-134.99, -127.2613) -> (-131.99, -124.2613) centre (-134.99, -124.2613) ccw
  line L376 (-149.6011, -141.8724) -> (-153.6011, -141.8724)
  arc A376 (-156.6011, -138.8724) -> (-153.6011, -141.8724) centre (-153.6011, -138.8724) ccw
  line L377 (-156.6011, -138.8724) -> (-156.6011, -134.8724)
  arc A377 (-153.6011, -131.8724) -> (-156.6011, -134.8724) centre (-153.6011, -134.8724) ccw
  line L378 (-153.6011, -131.8724) -> (-149.6011, -131.8724)
  arc A378 (-146.6011, -134.8724) -> (-149.6011, -131.8724) centre (-149.6011, -134.8724) ccw
  line L379 (-146.6011, -134.8724) -> (-146.6011, -138.8724)
  arc A379 (-149.6011, -141.8724) -> (-146.6011, -138.8724) centre (-149.6011, -138.8724) ccw
  line L380 (-164.2123, -39.5946) -> (-168.2123, -39.5946)
  arc A380 (-171.2123, -36.5946) -> (-168.2123, -39.5946) centre (-168.2123, -36.5946) ccw
  line L381 (-171.2123, -36.5946) -> (-171.2123, -32.5946)
  arc A381 (-168.2123, -29.5946) -> (-171.2123, -32.5946) centre (-168.2123, -32.5946) ccw
  line L382 (-168.2123, -29.5946) -> (-164.2123, -29.5946)
  arc A382 (-161.2123, -32.5946) -> (-164.2123, -29.5946) centre (-164.2123, -32.5946) ccw
  line L383 (-161.2123, -32.5946) -> (-161.2123, -36.5946)
  arc A383 (-164.2123, -39.5946) -> (-161.2123, -36.5946) centre (-164.2123, -36.5946) ccw
  line L384 (-91.1567, -156.4835) -> (-95.1567, -156.4835)
  arc A384 (-98.1567, -153.4835) -> (-95.1567, -156.4835) centre (-95.1567, -153.4835) ccw
  line L385 (-98.1567, -153.4835) -> (-98.1567, -149.4835)
  arc A385 (-95.1567, -146.4835) -> (-98.1567, -149.4835) centre (-95.1567, -149.4835) ccw
  line L386 (-95.1567, -146.4835) -> (-91.1567, -146.4835)
  arc A386 (-88.1567, -149.4835) -> (-91.1567, -146.4835) centre (-91.1567, -149.4835) ccw
  line L387 (-88.1567, -149.4835) -> (-88.1567, -153.4835)
  arc A387 (-91.1567, -156.4835) -> (-88.1567, -153.4835) centre (-91.1567, -153.4835) ccw
  line L388 (-76.5456, -127.2613) -> (-80.5456, -127.2613)
  arc A388 (-83.5456, -124.2613) -> (-80.5456, -127.2613) centre (-80.5456, -124.2613) ccw
  line L389 (-83.5456, -124.2613) -> (-83.5456, -120.2613)
  arc A389 (-80.5456, -117.2613) -> (-83.5456, -120.2613) centre (-80.5456, -120.2613) ccw
  line L390 (-80.5456, -117.2613) -> (-76.5456, -117.2613)
  arc A390 (-73.5456, -120.2613) -> (-76.5456, -117.2613) centre (-76.5456, -120.2613) ccw
  line L391 (-73.5456, -120.2613) -> (-73.5456, -124.2613)
  arc A391 (-76.5456, -127.2613) -> (-73.5456, -124.2613) centre (-76.5456, -124.2613) ccw
  line L392 (-164.2123, -54.2058) -> (-168.2123, -54.2058)
  arc A392 (-171.2123, -51.2058) -> (-168.2123, -54.2058) centre (-168.2123, -51.2058) ccw
  line L393 (-171.2123, -51.2058) -> (-171.2123, -47.2058)
  arc A393 (-168.2123, -44.2058) -> (-171.2123, -47.2058) centre (-168.2123, -47.2058) ccw
  line L394 (-168.2123, -44.2058) -> (-164.2123, -44.2058)
  arc A394 (-161.2123, -47.2058) -> (-164.2123, -44.2058) centre (-164.2123, -47.2058) ccw
  line L395 (-161.2123, -47.2058) -> (-161.2123, -51.2058)
  arc A395 (-164.2123, -54.2058) -> (-161.2123, -51.2058) centre (-164.2123, -51.2058) ccw
  line L396 (-164.2123, -98.0391) -> (-168.2123, -98.0391)
  arc A396 (-171.2123, -95.0391) -> (-168.2123, -98.0391) centre (-168.2123, -95.0391) ccw
  line L397 (-171.2123, -95.0391) -> (-171.2123, -91.0391)
  arc A397 (-168.2123, -88.0391) -> (-171.2123, -91.0391) centre (-168.2123, -91.0391) ccw
  line L398 (-168.2123, -88.0391) -> (-164.2123, -88.0391)
  arc A398 (-161.2123, -91.0391) -> (-164.2123, -88.0391) centre (-164.2123, -91.0391) ccw
  line L399 (-161.2123, -91.0391) -> (-161.2123, -95.0391)
  arc A399 (-164.2123, -98.0391) -> (-161.2123, -95.0391) centre (-164.2123, -95.0391) ccw
  arc A400 (-34.5946, -187.2342) -> (-13.5727, -166.2123) centre (-34.5946, -166.2123) ccw
  line L400 (-13.5727, -166.2123) -> (-13.5727, -34.5946)
  arc A401 (-13.5727, -34.5946) -> (-34.5946, -13.5727) centre (-34.5946, -34.5946) ccw
  line L401 (-34.5946, -13.5727) -> (-166.2123, -13.5727)
  arc A402 (-166.2123, -13.5727) -> (-187.2342, -34.5946) centre (-166.2123, -34.5946) ccw
  line L402 (-187.2342, -34.5946) -> (-187.2342, -166.2123)
  arc A403 (-187.2342, -166.2123) -> (-166.2123, -187.2342) centre (-166.2123, -166.2123) ccw
  line L403 (-166.2123, -187.2342) -> (-166.2123, -190.2123)
  line L404 (-166.2123, -190.2123) -> (-146.2123, -190.2123)
  line L405 (-146.2123, -190.2123) -> (-146.2123, -187.2342)
  line L406 (-146.2123, -187.2342) -> (-34.5946, -187.2342)
  line L407 (-180.0312, -39.5946) -> (-180.0312, -161.0946)
  line L408 (-20.1236, -39.5946) -> (-20.1236, -161.0946)
  line L409 (-184.5312, -39.5946) -> (-184.5312, -161.0946)
  arc A404 (-184.5312, -161.0946) -> (-175.5312, -161.0946) centre (-180.0312, -161.0946) ccw
  line L410 (-175.5312, -161.0946) -> (-175.5312, -39.5946)
  arc A405 (-175.5312, -39.5946) -> (-184.5312, -39.5946) centre (-180.0312, -39.5946) ccw
  line L411 (-180.0312, -39.5946) -> (-180.0312, -161.0946) construction
  line L412 (-24.6236, -39.5946) -> (-24.6236, -161.0946)
  arc A406 (-24.6236, -161.0946) -> (-15.6236, -161.0946) centre (-20.1236, -161.0946) ccw
  line L413 (-15.6236, -161.0946) -> (-15.6236, -39.5946)
  arc A407 (-15.6236, -39.5946) -> (-24.6236, -39.5946) centre (-20.1236, -39.5946) ccw
  line L414 (-20.1236, -39.5946) -> (-20.1236, -161.0946) construction
  line L415 (-39.7123, -175.7925) -> (-161.2123, -175.7925)
  arc A408 (-161.2123, -175.7925) -> (-161.2123, -184.7925) centre (-161.2123, -180.2925) ccw
  line L416 (-161.2123, -184.7925) -> (-39.7123, -184.7925)
  arc A409 (-39.7123, -184.7925) -> (-39.7123, -175.7925) centre (-39.7123, -180.2925) ccw
  line L417 (-39.7123, -180.2925) -> (-161.2123, -180.2925) construction
  line L418 (-161.2123, -24.8849) -> (-39.7123, -24.8849)
  arc A410 (-39.7123, -24.8849) -> (-39.7123, -15.8849) centre (-39.7123, -20.3849) ccw
  line L419 (-39.7123, -15.8849) -> (-161.2123, -15.8849)
  arc A411 (-161.2123, -15.8849) -> (-161.2123, -24.8849) centre (-161.2123, -20.3849) ccw
  line L420 (-161.2123, -20.3849) -> (-39.7123, -20.3849) construction
  dimension "d139" = 9
  dimension "d140" = 9
  dimension "d141" = 9
  dimension "d142" = 9
  constraint perpendicular L262 L407
  constraint perpendicular L234 L408
  constraint tangent L409 A404
  constraint tangent A404 L410
  constraint parallel L409 L410
  constraint tangent L410 A405
  constraint tangent L409 A405
  constraint coincident L407.end A404.centre
  constraint parallel L407 L411
  constraint coincident L407.start A405.centre
  constraint tangent L412 A406
  constraint tangent A406 L413
  constraint parallel L412 L413
  constraint tangent L413 A407
  constraint tangent L412 A407
  constraint coincident L408.end A406.centre
  constraint parallel L408 L414
  constraint coincident L408.start A407.centre
  constraint tangent L415 A408
  constraint tangent A408 L416
  constraint parallel L415 L416
  constraint tangent L416 A409
  constraint tangent L415 A409
  constraint perpendicular L263 L417
  constraint tangent L418 A410
  constraint tangent A410 L419
  constraint parallel L418 L419
  constraint tangent L419 A411
  constraint tangent L418 A411
  constraint perpendicular L281 L420
  measures "d139" diameter of A404
  measures "d140" diameter of A406
  measures "d141" diameter of A408
  measures "d142" diameter of A410
extrude "Extrude31" cut sketch "Sketch13" against normal blind 15 contours L409 A404 L410 A405 | L412 A406 L413 A407 | L415 A408 L416 A409 | L418 A410 L419 A411 bodies 11
fillet "Fillet2" radius 2 4 edges at (18.7451, 172.3597, 26) (150.3627, 172.3597, 26) (150.3627, 40.7421, 26) (18.7451, 40.7421, 26) on bodies 12
extrude "Extrude32" cut sketch "Sketch12" along normal blind 60 contours A12 L17 A13 L18 A14 L19 A15 L20 | A16 L21 A17 L22 A18 L23 A19 L24 | A20 L25 A21 L26 A22 L27 A23 L28 | A24 L29 A25 L30 A26 L31 A27 L32 | A28 L33 A29 L34 A30 L35 A31 L36 | A32 L37 A33 L38 A34 L39 A35 L40 | A52 L57 A53 L58 A54 L59 A55 L60 | A56 L61 A57 L62 A58 L63 A59 L64 | A60 L65 A61 L66 A62 L67 A63 L68 | A64 L69 A65 L70 A66 L71 A67 L72 | A68 L73 A69 L74 A70 L75 A71 L76 | A72 L77 A73 L78 A74 L79 A75 L80 | A84 L89 A85 L90 A86 L91 A87 L92 | A88 L93 A89 L94 A90 L95 A91 L96 | A92 L97 A93 L98 A94 L99 A95 L100 | A96 L101 A97 L102 A98 L103 A99 L104 | A100 L105 A101 L106 A102 L107 A103 L108 | A104 L109 A105 L110 A106 L111 A107 L112 | A108 L113 A109 L114 A110 L115 A111 L116 | A112 L117 A113 L118 A114 L119 A115 L120 | A116 L121 A117 L122 A118 L123 A119 L124 | A120 L125 A121 L126 A122 L127 A123 L128 | A124 L129 A125 L130 A126 L131 A127 L132 | A128 L133 A129 L134 A130 L135 A131 L136 | A132 L137 A133 L138 A134 L139 A135 L140 | A136 L141 A137 L142 A138 L143 A139 L144 | A140 L145 A141 L146 A142 L147 A143 L148 | A144 L149 A145 L150 A146 L151 A147 L152 | A148 L153 A149 L154 A150 L155 A151 L156 | A152 L157 A153 L158 A154 L159 A155 L160 | A156 L161 A157 L162 A158 L163 A159 L164 | A160 L165 A161 L166 A162 L167 A163 L168 | A164 L169 A165 L170 A166 L171 A167 L172 | A168 L173 A169 L174 A170 L175 A171 L176 | A172 L177 A173 L178 A174 L179 A175 L180 | A176 L181 A177 L182 A178 L183 A179 L184 | A180 L185 A181 L186 A182 L187 A183 L188 | A184 L189 A185 L190 A186 L191 A187 L192 | A188 L193 A189 L194 A190 L195 A191 L196 | A192 L197 A193 L198 A194 L199 A195 L200 | A196 L201 A197 L202 A198 L203 A199 L204 | A200 L205 A201 L206 A202 L207 A203 L208 | A204 L209 A205 L210 A206 L211 A207 L212 | A208 L213 A209 L214 A210 L215 A211 L216 | A212 L217 A213 L218 A214 L219 A215 L220 | A216 L221 A217 L222 A218 L223 A219 L224 | A220 L225 A221 L226 A222 L227 A223 L228 | A224 L229 A225 L230 A226 L231 A227 L232 | A228 L233 A229 L234 A230 L235 A231 L236 | A232 L237 A233 L238 A234 L239 A235 L240 | A236 L241 A237 L242 A238 L243 A239 L244 | A240 L245 A241 L246 A242 L247 A243 L248 | A244 L249 A245 L250 A246 L251 A247 L252 | A248 L253 A249 L254 A250 L255 A251 L256 | A252 L257 A253 L258 A254 L259 A255 L260 | A256 L261 A257 L262 A258 L263 A259 L264 | A260 L265 A261 L266 A262 L267 A263 L268 | A264 L269 A265 L270 A266 L271 A267 L272 | A268 L273 A269 L274 A270 L275 A271 L276 | A272 L277 A273 L278 A274 L279 A275 L280 | A276 L281 A277 L282 A278 L283 A279 L284 | A280 L285 A281 L286 A282 L287 A283 L288 | A284 L289 A285 L290 A286 L291 A287 L292 | A288 L293 A289 L294 A290 L295 A291 L296 | A292 L297 A293 L298 A294 L299 A295 L300 | A296 L301 A297 L302 A298 L303 A299 L304 | A300 L305 A301 L306 A302 L307 A303 L308 | A304 L309 A305 L310 A306 L311 A307 L312 | A308 L313 A309 L314 A310 L315 A311 L316 | A312 L317 A313 L318 A314 L319 A315 L320 | A316 L321 A317 L322 A318 L323 A319 L324 | A320 L325 A321 L326 A322 L327 A323 L328 | A332 L337 A333 L338 A334 L339 A335 L340 | A336 L341 A337 L342 A338 L343 A339 L344 | A340 L345 A341 L346 A342 L347 A343 L348 | A344 L349 A345 L350 A346 L351 A347 L352 | A348 L353 A349 L354 A350 L355 A351 L356 | A352 L357 A353 L358 A354 L359 A355 L360 | A372 L377 A373 L378 A374 L379 A375 L380 | A376 L381 A377 L382 A378 L383 A379 L384 | A380 L385 A381 L386 A382 L387 A383 L388 | A384 L389 A385 L390 A386 L391 A387 L392 | A388 L393 A389 L394 A390 L395 A391 L396 | A392 L397 A393 L398 A394 L399 A395 L400 bodies 12
extrude "Extrude33" cut 4 faces at (184.4711, 165.2186, 8) (52.7977, 164.4734, 8) (52.8535, 33.601, 8) (184.4711, 33.601, 8) along direction (0, 0, 1) blind 5 on bodies 12 bodies 12
copy_body "CopyPasteBodies2" bodies 12 makes body 13
move_body "Move8" bodies 13 to x (1, 0, 0) y (0, 1, 0) z (0, 0, 1) at (0, 0, 0)
move_body "Move7" bodies 12 to x (-1, 0, 0) y (0, 1, 0) z (0, 0, -1) at (11.1893, 0, 56)
hidden bodies 1 10 13
equation "d1 = d2"
equation "d14 = ( 15.88 / 2 ) * 1 mm"
equation "d15 = ( -15.88 / 2 ) * 1 mm"
equation "d16 = ( 13.5 / 2 ) * 1 mm"
equation "d17 = ( -13.5 / 2 ) * 1 mm"
named bodies: "DownPart", "TopPart", "TopPart (1)"
